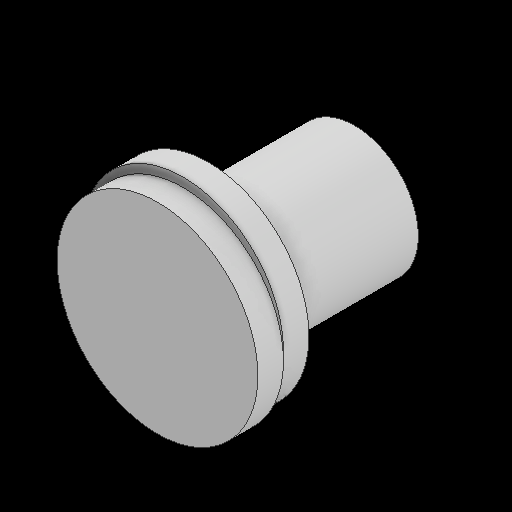
# Autodesk Inventor part: input_shaft
Saved by Autodesk Inventor 2026 (Build 300175050, 175E)
## iProperties
Created: 2026-06-07
Part Number: input_shaft
Material: 일반
Document SubType Name: Modeling
Designer: iamma
Density: 1 g/cm^3
Appearance: 기본값
Author: iamma
Autodesk Inventor part; units mm, degrees
ref_plane "YZ Plane" through (0, 0, 0) normal (1, 0, 0) x (0, 1, 0)
ref_plane "XZ Plane" through (0, 0, 0) normal (0, 1, 0) x (-1, 0, 0)
ref_plane "XY Plane" through (0, 0, 0) normal (0, 0, 1) x (1, 0, 0)
sketch "스케치1" plane through (0, 0, 0) normal (0, 0, 1) x (1, 0, 0)
  circle A0 centre (0, 0) radius 17.5
  dimension "d0" = 35
  constraints: 1 centre point, 1 coincident
  measures "d0" diameter of A0
extrude "돌출1" add sketch "스케치1" along normal blind 40
sketch "스케치2" plane through (0, 0, 40) normal (0, 0, 1) x (1, 0, 0)
  circle A0 centre (0, 1.233) radius 27.5
  point P0 (0, 0)
  dimension "d3" = 55
  dimension "d4" = 1.233
  constraints: 1 centre point, 1 vertical alignment
  measures "d3" diameter of A0
  measures "d4" distance of point (0, 0) A0.centre
extrude "돌출2" add sketch "스케치2" along normal blind 7
sketch "스케치3" plane through (0, 1.233, 47) normal (0, 0, 1) x (1, 0, 0)
  circle A0 centre (0, -1.233) radius 17.5 construction
  circle A1 centre (0, -1.233) radius 17.5 construction
  circle A2 centre (0, -1.233) radius 17.5 construction
  circle A3 centre (0, -2.466) radius 27.5
  dimension "d7" = 1.233
  dimension "d8" = 55
  constraints: 1 centre point, 1 vertical alignment
  measures "d7" distance of A3.centre point (0, -1.233)
  measures "d8" diameter of A3
extrude "돌출3" add sketch "스케치3" along normal blind 7
